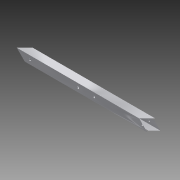
# Autodesk Inventor part: 1x1 horizontal support
Saved by Autodesk Inventor 2015 SP1 (Build 190203100, 203)
## iProperties
Created: 2015-01-18
Part Number: 1x1 horizontal support
Material: Aluminum 6061
Document SubType Name: Modeling
Designer: Jarod
Density: 2.7 g/cm^3
Appearance: Aluminum - Flat
Author: Jarod
Autodesk Inventor part; units mm, degrees
ref_plane "YZ Plane" through (0, 0, 0) normal (1, 0, 0) x (0, 1, 0)
ref_plane "XZ Plane" through (0, 0, 0) normal (0, 1, 0) x (-1, 0, 0)
ref_plane "XY Plane" through (0, 0, 0) normal (0, 0, 1) x (1, 0, 0)
sketch "Sketch1" plane through (0, 0, 0) normal (1, 0, 0) x (0, 1, 0)
  line L0 (0, 0) -> (-25.4, 0)
  line L1 (-25.4, 0) -> (-25.4, 25.4)
  line L2 (-25.4, 25.4) -> (0, 25.4)
  line L3 (0, 25.4) -> (0, 0)
  line L4 (-3.175, 3.175) -> (-22.225, 3.175)
  line L5 (-22.225, 3.175) -> (-22.225, 22.225)
  line L6 (-22.225, 22.225) -> (-3.175, 22.225)
  line L7 (-3.175, 22.225) -> (-3.175, 3.175)
  dimension "d0" = 25.4
  dimension "d1" = 25.4
  dimension "d2" = 19.05
  dimension "d3" = 19.05
  dimension "d4" = 3.175
  dimension "d5" = 3.175
  constraints: 16 end point, 4 parallel, 2 horizontal, 2 perpendicular
  measures "d0" distance of L1.end L2.end
  measures "d1" distance of L0.end L1.end
  measures "d2" distance of L5.end L6.end
  measures "d3" distance of L4.end L5.end
  measures "d4" distance between parallel lines of L0 L4
  measures "d5" distance between parallel lines of L3 L7
extrude "Extrusion1" add sketch "Sketch1" along normal blind 546.1
sketch "Sketch2" plane through (0, -25.4, 25.4) normal (0, 0, 1) x (1, 0, 0)
  line L0 (0, 0) -> (0, 25.4) projected
  line L1 (0, 0) -> (546.1, 0) projected
  line L2 (546.1, 25.4) -> (546.1, 0) projected
  line L3 (0, 25.4) -> (546.1, 25.4) projected
  point P0 (12.7, 12.7)
  point P1 (533.4, 12.7)
  dimension "d8" = 12.7
  dimension "d9" = 12.7
  dimension "d10" = 12.7
  dimension "d11" = 12.7
  measures "d8" distance from line of L2 point (533.4, 12.7)
  measures "d9" distance from line of L1 point (533.4, 12.7)
  measures "d10" distance from line of L0 point (12.7, 12.7)
  measures "d11" distance from line of L3 point (12.7, 12.7)
hole "Hole1" at (12.7, -12.7, 25.4) at (533.4, -12.7, 25.4) direction (0, 0, -1) diameter 6.35 end through all
sketch "Sketch3" plane through (0, -25.4, 25.4) normal (0, 0, 1) x (1, 0, 0)
  circle A0 centre (12.7, 12.7) radius 3.175 projected
  circle A1 centre (533.4, 12.7) radius 3.175 projected
  line L0 (0, 0) -> (0, 25.4) projected
  line L1 (0, 0) -> (546.1, 0) projected
  line L2 (546.1, 25.4) -> (546.1, 0) projected
  line L3 (0, 25.4) -> (546.1, 25.4) projected
  point P0 (247.65, 12.7)
  point P1 (298.45, 12.7)
  dimension "d19" = 247.65
  dimension "d20" = 247.65
  dimension "d21" = 12.7
  dimension "d22" = 12.7
  measures "d19" distance from line of L0 point (247.65, 12.7)
  measures "d20" distance from line of L2 point (298.45, 12.7)
  measures "d21" distance from line of L1 point (298.45, 12.7)
  measures "d22" distance from line of L1 point (247.65, 12.7)
hole "Hole2" at (247.65, -12.7, 25.4) at (298.45, -12.7, 25.4) direction (0, 0, -1) diameter 6.35 end through all
sketch "Sketch4" plane through (0, -25.4, 25.4) normal (0, 0, 1) x (1, 0, 0)
  circle A0 centre (247.65, 12.7) radius 3.175 projected
  circle A1 centre (298.45, 12.7) radius 3.175 projected
  circle A2 centre (12.7, 12.7) radius 3.175 projected
  circle A3 centre (533.4, 12.7) radius 3.175 projected
  line L0 (0, 0) -> (0, 25.4) projected
  line L1 (0, 0) -> (546.1, 0) projected
  line L2 (546.1, 25.4) -> (546.1, 0) projected
  line L3 (0, 25.4) -> (546.1, 25.4) projected
  point P0 (38.1, 12.7)
  point P1 (508, 12.7)
  dimension "d30" = 38.1
  dimension "d31" = 12.7
  dimension "d32" = 12.7
  dimension "d33" = 38.1
  measures "d30" distance from line of point (38.1, 12.7) L0
  measures "d31" distance from line of L1 point (38.1, 12.7)
  measures "d32" distance from line of L1 point (508, 12.7)
  measures "d33" distance from line of L2 point (508, 12.7)
hole "Hole3" at (38.1, -12.7, 25.4) at (508, -12.7, 25.4) direction (0, 0, -1) diameter 4.7625 end through all
sketch "Sketch7" plane through (0, -25.4, 25.4) normal (0, 0, 1) x (1, 0, 0)
  circle A0 centre (38.1, 12.7) radius 2.3813 projected
  circle A1 centre (508, 12.7) radius 2.3813 projected
  line L0 (0, 0) -> (546.1, 0) projected
  circle A2 centre (38.1, 12.7) radius 3.175
  circle A3 centre (95.25, 12.7) radius 3.175
  circle A4 centre (508, 12.7) radius 2.3813 projected
  circle A5 centre (508, 12.7) radius 3.175
  circle A6 centre (450.85, 12.7) radius 3.175
  dimension "d65" = 6.35
  dimension "d66" = 6.35
  dimension "d67" = 12.7
  dimension "d68" = 57.15
  dimension "d69" = 6.35
  dimension "d70" = 6.35
  dimension "d71" = 12.7
  dimension "d72" = 57.15
  constraints: 4 centre point, 2 coincident
  measures "d65" diameter of A2
  measures "d66" diameter of A3
  measures "d67" distance from line of A3.centre L0
  measures "d68" distance of A0.centre A3.centre
  measures "d69" diameter of A5
  measures "d70" diameter of A6
  measures "d71" distance from line of L0 A6.centre
  measures "d72" distance of A1.centre A6.centre
extrude "Extrusion2" cut sketch "Sketch7" against normal blind 25.4
sketch "Sketch8" plane through (0, 0, 0) normal (-1, 0, 0) x (0, 0, 1)
  line L0 (22.225, -22.225) -> (3.175, -22.225) projected
  line L1 (3.175, -22.225) -> (3.175, -3.175) projected
  line L2 (3.175, -3.175) -> (22.225, -3.175) projected
  line L3 (22.225, -3.175) -> (22.225, -22.225) projected
  line L4 (0, 0) -> (0, -25.4) projected
  line L5 (0, -25.4) -> (25.4, -25.4) projected
  line L6 (25.4, -25.4) -> (25.4, 0) projected
  line L7 (25.4, 0) -> (0, 0) projected
extrude "Extrusion3" cut sketch "Sketch8" against normal blind 25.4
sketch "Sketch9" plane through (546.1, 0, 0) normal (1, 0, 0) x (0, 0, -1)
  line L0 (-3.175, -22.225) -> (-22.225, -22.225) projected
  line L1 (-22.225, -22.225) -> (-22.225, -3.175) projected
  line L2 (-22.225, -3.175) -> (-3.175, -3.175) projected
  line L3 (-3.175, -3.175) -> (-3.175, -22.225) projected
  line L4 (0, -25.4) -> (0, 0) projected
  line L5 (0, 0) -> (-25.4, 0) projected
  line L6 (-25.4, 0) -> (-25.4, -25.4) projected
  line L7 (-25.4, -25.4) -> (0, -25.4) projected
extrude "Extrusion4" cut sketch "Sketch9" against normal blind 25.4
body "Solid1"
